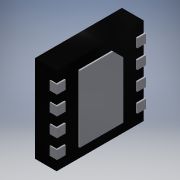
# Autodesk Inventor part: MAX30205
Saved by Autodesk Inventor 2018.3 (Build 223284000, 284)
## iProperties
Created: 2021-06-02
Part Number: MAX30205
Material: Genérico
Document SubType Name: Modeling
Designer: laguerre
Density: 8.47 g/cm^3
Appearance: Negro
Author: laguerre
Autodesk Inventor part; units mm, degrees
note: some values were not read from the file. Chosen so that the rebuilt part matches the saved one: direction of "Repujado1".
ref_plane "YZ Plane" through (0, 0, 0) normal (1, 0, 0) x (0, 1, 0)
ref_plane "XZ Plane" through (0, 0, 0) normal (0, 1, 0) x (-1, 0, 0)
ref_plane "XY Plane" through (0, 0, 0) normal (0, 0, 1) x (1, 0, 0)
sketch "Boceto39" plane through (0, 0, 0) normal (0, 0, 1) x (1, 0, 0)
  line L0 (-1.5, 1.5) -> (1.5, 1.5)
  line L1 (1.5, 1.5) -> (1.5, -1.5)
  line L2 (1.5, -1.5) -> (-1.5, -1.5)
  line L3 (-1.5, -1.5) -> (-1.5, 1.5)
  point P0 (0, 0)
  point P1 (0, 1.5)
  point P2 (-1.5, 0)
  dimension "d373" = 3
  dimension "d374" = 3
  constraints: 8 end point, 2 midpoint, 2 parallel, 1 horizontal, 1 horizontal alignment, 1 perpendicular, 1 vertical alignment
  measures "d373" distance of L0.start L0.end
  measures "d374" distance of L2.end L0.start
extrude "Extrusión13" add sketch "Boceto39" along normal blind 0.75
sketch "Boceto40" plane through (0, 0, 0.75) normal (0, 0, 1) x (1, 0, 0)
  circle A0 centre (-1.1, 1.1) radius 0.15
  line L0 (-1.5, 1.5) -> (-1.5, -1.5) projected
  line L1 (1.5, 1.5) -> (-1.5, 1.5) projected
  point P0 (0, 0)
  dimension "d377" = 0.4
  dimension "d378" = 0.4
  dimension "d379" = 0.3
  constraints: 1 centre point
  measures "d377" distance from line of L0 A0.centre
  measures "d378" distance from line of A0.centre L1
  measures "d379" diameter of A0
emboss "Repujado1" sketch "Boceto40" operation cut depth 0.001 direction (0, 0, -1)
sketch "Boceto41" plane through (0, 0, 0) normal (0, 0, -1) x (-1, 0, 0)
  line L0 (1.235, 1.125) -> (1.535, 1.125)
  line L1 (1.535, 1.125) -> (1.535, 0.825)
  line L2 (1.535, 0.825) -> (1.235, 0.825)
  line L3 (1.235, 0.825) -> (1.235, 1.125)
  line L4 (1.235, 0.475) -> (1.535, 0.475)
  line L5 (1.535, 0.475) -> (1.535, 0.175)
  line L6 (1.535, 0.175) -> (1.235, 0.175)
  line L7 (1.235, 0.175) -> (1.235, 0.475)
  line L8 (1.235, -0.175) -> (1.535, -0.175)
  line L9 (1.535, -0.175) -> (1.535, -0.475)
  line L10 (1.535, -0.475) -> (1.235, -0.475)
  line L11 (1.235, -0.475) -> (1.235, -0.175)
  line L12 (1.535, -0.825) -> (1.235, -0.825)
  line L13 (1.235, -0.825) -> (1.235, -1.125)
  line L14 (1.235, -1.125) -> (1.535, -1.125)
  line L15 (1.535, -1.125) -> (1.535, -0.825)
  line L16 (-1.535, 1.125) -> (-1.235, 1.125)
  line L17 (-1.235, 1.125) -> (-1.235, 0.825)
  line L18 (-1.235, 0.825) -> (-1.535, 0.825)
  line L19 (-1.535, 0.825) -> (-1.535, 1.125)
  line L20 (-1.535, 0.475) -> (-1.235, 0.475)
  line L21 (-1.235, 0.475) -> (-1.235, 0.175)
  line L22 (-1.235, 0.175) -> (-1.535, 0.175)
  line L23 (-1.535, 0.175) -> (-1.535, 0.475)
  line L24 (-1.535, -0.175) -> (-1.235, -0.175)
  line L25 (-1.235, -0.175) -> (-1.235, -0.475)
  line L26 (-1.235, -0.475) -> (-1.535, -0.475)
  line L27 (-1.535, -0.475) -> (-1.535, -0.175)
  line L28 (-1.235, -0.825) -> (-1.535, -0.825)
  line L29 (-1.535, -0.825) -> (-1.535, -1.125)
  line L30 (-1.535, -1.125) -> (-1.235, -1.125)
  line L31 (-1.235, -1.125) -> (-1.235, -0.825)
  line L32 (-0.75, 1.15) -> (0.4, 1.15)
  line L33 (0.75, 0.8) -> (0.75, -1.15)
  line L34 (0.75, -1.15) -> (-0.75, -1.15)
  line L35 (-0.75, -1.15) -> (-0.75, 1.15)
  line L36 (0.4, 1.15) -> (0.75, 0.8)
  line L37 (-1.5, 1.5) -> (-1.5, -1.5) projected
  line L38 (1.5, -1.5) -> (1.5, 1.5) projected
  point P0 (0, 0)
  point P1 (-1.235, 0.975)
  point P2 (1.235, 0.975)
  point P3 (1.235, 0.325)
  point P4 (-1.235, 0.325)
  point P5 (-1.235, -0.325)
  point P6 (1.235, -0.325)
  point P7 (1.235, -0.975)
  point P8 (-1.235, -0.975)
  point P9 (-0.75, 0)
  point P10 (0, -1.15)
  dimension "d391" = 0.65
  dimension "d394" = 0.65
  dimension "d407" = 0.325
  dimension "d408" = 0.035
  dimension "d409" = 0.035
  dimension "d410" = 0.3
  dimension "d411" = 0.3
  dimension "d412" = 0.65
  dimension "d413" = 1.5
  dimension "d414" = 0.35
  dimension "d415" = 0.35
  dimension "d416" = 2.3
  constraints: 74 end point, 18 parallel, 13 equal length, 10 midpoint, 9 horizontal, 9 perpendicular, 5 collinear, 5 horizontal alignment, 2 point on line, 1 vertical alignment
  measures "d391" distance of point (-1.235, 0.975) point (-1.235, 0.325)
  measures "d394" distance of point (-1.235, -0.325) point (-1.235, -0.975)
  measures "d407" vertical distance of point (0, 0) point (-1.235, -0.325)
  measures "d408" distance between parallel lines of L37 L19
  measures "d409" distance between parallel lines of L38 L1
  measures "d410" distance of L19.start L19.end
  measures "d411" distance of L0.start L0.end
  measures "d412" distance of point (-1.235, -0.325) point (-1.235, 0.325)
  measures "d413" distance between parallel lines of L33 L35
  measures "d414" horizontal distance of L32.end L33.start
  measures "d415" horizontal distance of L32.end L33.start
  measures "d416" distance between parallel lines of L32 L34
extrude "Extrusión14" add sketch "Boceto41" along normal blind 0.05 and the other way blind 0.203
